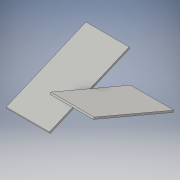
# Autodesk Inventor part: SeeSaw
Saved by Autodesk Inventor 2016 (Build 200138000, 138)
## iProperties
Created: 2016-01-10
Part Number: SeeSaw
Material: Generic
Document SubType Name: Modeling
Designer: hartc3
Density: 1 g/cm^3
Appearance: Default
Author: hartc3
Autodesk Inventor part; units mm, degrees
ref_plane "YZ Plane" through (0, 0, 0) normal (1, 0, 0) x (0, 1, 0)
ref_plane "XZ Plane" through (0, 0, 0) normal (0, 1, 0) x (-1, 0, 0)
ref_plane "XY Plane" through (0, 0, 0) normal (0, 0, 1) x (1, 0, 0)
sketch "Sketch1" plane through (0, 0, 0) normal (1, 0, 0) x (0, 1, 0)
  line L0 (0, 0) -> (238.1897, -561.1398)
  line L1 (0, 0) -> (0, -331.1226) construction
  line L2 (0, 0) -> (11.6904, 4.9623)
  line L3 (11.6904, 4.9623) -> (249.8801, -556.1775)
  line L4 (249.8801, -556.1775) -> (238.1897, -561.1398)
  dimension "d0" = 609.6
  dimension "d2" = 23
  dimension "d3" = 12.7
  constraints: 10 end point, 2 perpendicular, 1 parallel, 1 vertical
  measures "d0" distance of L0.start L0.end
  measures "d2" angle of L0 L1
  measures "d3" distance of L0.start L2.end
extrude "Extrusion1" add sketch "Sketch1" along normal blind 304.8
sketch "Sketch2" plane through (304.8, 0, 0) normal (1, 0, 0) x (0, 0, -1)
  line L0 (0, 0) -> (561.1398, 238.1897) projected
  line L1 (561.1398, 0) -> (0, 238.1897)
  line L2 (561.1398, 0) -> (392.1686, 0) construction
  line L3 (4.9623, 249.8801) -> (566.102, 11.6904)
  line L4 (4.9623, 249.8801) -> (0, 238.1897)
  line L5 (561.1398, 0) -> (566.102, 11.6904)
  dimension "d6" = 23
  dimension "d7" = 12.7
  dimension "d8" = 609.6
  constraints: 10 end point, 2 perpendicular, 1 horizontal, 1 horizontal alignment, 1 vertical alignment
  measures "d6" angle of L2 L1
  measures "d7" distance between parallel lines of L1 L3
  measures "d8" distance of L1.start L1.end
extrude "Extrusion2" add sketch "Sketch2" along normal blind 304.8
body "Solid1"
